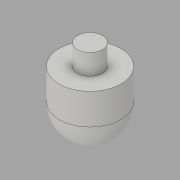
# Autodesk Inventor part: 2-2-7
Saved by Autodesk Inventor 2019 (Build 230136000, 136)
## iProperties
Created: 2020-11-06
Part Number: 2-2-7
Material: 一般
Document SubType Name: Modeling
Designer: Sugar
Density: 1 g/cm^3
Appearance: 預設
Author: Sugar
Autodesk Inventor part; units mm, degrees
ref_plane "YZ Plane" through (0, 0, 0) normal (1, 0, 0) x (0, 1, 0)
ref_plane "XZ Plane" through (0, 0, 0) normal (0, 1, 0) x (-1, 0, 0)
ref_plane "XY Plane" through (0, 0, 0) normal (0, 0, 1) x (1, 0, 0)
sketch "草圖1" plane through (0, 0, 0) normal (0, 0, 1) x (1, 0, 0)
  line L0 (-6, 0) -> (0, 0)
  line L1 (0, 0) -> (0, -10)
  line L2 (0, -10) -> (-6, -10)
  line L3 (-6, -10) -> (-6, 0)
  line L4 (-15, -10) -> (0, -10)
  line L5 (0, -10) -> (0, -25)
  line L6 (0, -25) -> (-15, -25)
  line L7 (-15, -25) -> (-15, -10)
  arc A0 (-15, -25) -> (0, -40) centre (0, -25) ccw
  line L8 (0, -25) -> (0, -40)
  dimension "d0" = 6
  dimension "d1" = 15
  dimension "d2" = 10
  dimension "d3" = 25
  constraints: 18 end point, 4 parallel, 2 horizontal, 2 perpendicular, 2 point on circle, 1 centre point, 1 coincident, 1 line through centre, 1 tangent, 1 vertical
  measures "d0" distance of L0.start L0.end
  measures "d1" distance between parallel lines of L5 L7
  measures "d2" distance of L2.end L0.start
  measures "d3" distance between parallel lines of L6 L0
revolve "迴轉1" add sketch "草圖1" angle 360 about axis through (0, -10, 0) along (0, -1, 0)
